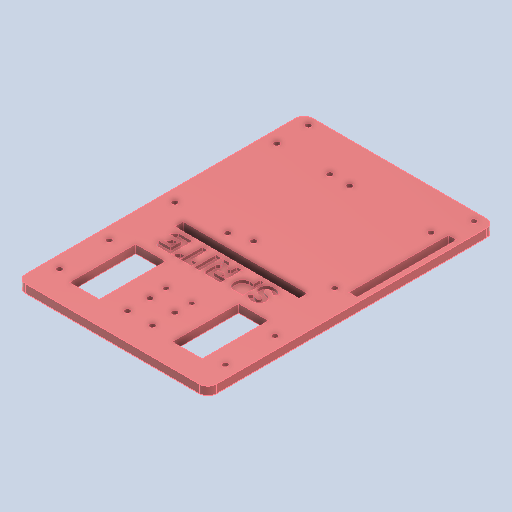
# Autodesk Inventor part: top plate modified
Saved by Autodesk Inventor 2025.1 (Build 291241020, 241B)
## iProperties
Created: 2024-03-20
Part Number: top plate modified
Material: Generic
Document SubType Name: Modeling
Designer: david
Density: 1 g/cm^3
Appearance: Smooth - Red
Description: Top Plate
Author: david
Autodesk Inventor part; units mm, degrees
ref_plane "YZ Plane" through (0, 0, 0) normal (1, 0, 0) x (0, 1, 0)
ref_plane "XZ Plane" through (0, 0, 0) normal (0, 1, 0) x (-1, 0, 0)
ref_plane "XY Plane" through (0, 0, 0) normal (0, 0, 1) x (1, 0, 0)
sketch "Sketch1" plane through (0, 0, 0) normal (0, 1, 0) x (-1, 0, 0)
  line L0 (57.5, -173) -> (57.5, -173) construction
  line L1 (-57.5, -173) -> (-57.5, 0) construction
  line L2 (-57.5, 0) -> (57.5, 0)
  line L3 (57.5, 0) -> (57.5, -173) construction
  line L4 (80.5, 0) -> (-80.5, 0) construction
  line L5 (0, -207.6) -> (0, 34.6) construction
  line L6 (57.5, -173) -> (-57.5, -173)
  line L7 (-57.5, -173) -> (-57.5, -173) construction
  line L8 (57.5, 0) -> (-55.1767, 0)
  line L9 (57.5, -40) -> (-57.5, -40) construction
  line L10 (-57.5, -40) -> (-57.5, 0)
  line L11 (-57.5, 0) -> (57.5, 0)
  line L12 (57.5, 0) -> (57.5, -40)
  line L13 (-57.5, -173) -> (-57.5, -40)
  line L14 (57.5, -173) -> (57.5, -40)
  point P0 (0, 0)
  dimension "width" = 115
  dimension "Length" = 173
  dimension "d2" = 115
  dimension "d112" = 40
  constraints: 26 end point, 6 parallel, 5 horizontal, 4 perpendicular, 1 collinear, 1 point on line, 1 symmetric about line, 1 vertical alignment, 1 other
  measures "width" distance of L1.end L2.end
  measures "Length" distance of L1.start L1.end
  measures "d2" distance of L6.end L0.end
  measures "d112" distance between parallel lines of L2 L9
extrude "Base" add sketch "Sketch1" against normal blind 5
sketch "Sketch11" plane through (0, 0, 0) normal (0, 1, 0) x (1, 0, 0)
  line L0 (0, 207.6) -> (0, -34.6) construction
  line L1 (-57.5, 0) -> (57.5, 0) construction
  line L2 (57.5, 173) -> (-57.5, 173) projected
  line L3 (-50, 18) -> (50, 18) construction
  line L4 (50, 18) -> (50, 48) construction
  line L5 (50, 48) -> (-50, 48) construction
  line L6 (-50, 48) -> (-50, 18) construction
  point P0 (0, 0)
  point P1 (50, 168)
  point P2 (-50, 168)
  dimension "d91" = 18
  dimension "d92" = 50
  dimension "d93" = 5
  dimension "d94" = 50
  dimension "d113" = 30
  constraints: 8 end point, 2 coincident, 2 parallel, 2 symmetric about line, 1 horizontal, 1 perpendicular, 1 vertical alignment
  measures "d91" distance from line of L1 point (50, 18)
  measures "d92" distance from line of point (50, 18) L0
  measures "d93" distance from line of L2 point (50, 168)
  measures "d94" distance from line of L0 point (50, 168)
  measures "d113" distance of L3.end L4.end
hole "Mounting Holes" at (50, 0, -18) at (-50, 0, -18) at (50, 0, -168) at (-50, 0, -168) at (-50, 0, -48) at (50, 0, -48) direction (0, -1, 0) diameter 3.4 depth 6
fillet "Fillet1" radius 5 4 edges at (-57.5, -2.5, 0) (57.5, -2.5, -173) (-57.5, -2.5, -173) (57.5, -2.5, 0)
sketch "Sketch12" plane through (0, 0, 0) normal (0, 1, 0) x (1, 0, 0)
  line L0 (-6, 149) -> (43, 149) construction
  line L1 (43, 149) -> (43, 91) construction
  line L2 (43, 91) -> (-6, 91) construction
  line L3 (-6, 91) -> (-6, 149) construction
  line L4 (-57.5, 168) -> (-57.5, 5) projected
  line L5 (0, 207.6) -> (0, -34.6) projected
  line L6 (-52.5, 0) -> (52.5, 0) projected
  circle A0 centre (-50, 48) radius 1.7 projected
  line L7 (52.5, 173) -> (-52.5, 173) projected
  circle A1 centre (50, 48) radius 1.7 projected
  circle A2 centre (50, 168) radius 1.7 projected
  point P0 (0, 0)
  point P1 (0, 0)
  point P2 (52.2987, 0)
  point P3 (-57.5, 40)
  point P4 (0, 0)
  dimension "d104" = 58
  dimension "d263" = 24
  dimension "d266" = 49
  dimension "d267" = 7
  constraints: 8 end point, 1 horizontal, 1 midpoint, 1 parallel, 1 perpendicular, 1 vertical
  measures "d104" distance of L0.end L1.end
  measures "d263" distance between parallel lines of L7 L0
  measures "d266" distance of L1.end L2.end
  measures "d267" distance from line of L1 A2.centre
hole "RasPi Mounting Holes" at (-6, 0, -149) at (43, 0, -149) at (43, 0, -91) at (-6, 0, -91) direction (0, -1, 0) diameter 3.4 depth 6
sketch "Sketch15" plane through (0, 0, 0) normal (0, 1, 0) x (1, 0, 0)
  line L0 (-18, 149) -> (-18, 87.5) construction
  line L1 (-18, 87.5) -> (-50, 87.5) construction
  line L2 (-50, 87.5) -> (-50, 149) construction
  line L3 (-50, 149) -> (-18, 149) construction
  line L4 (-52.5, 0) -> (52.5, 0) projected
  circle A0 centre (43, 149) radius 1.7 projected
  circle A1 centre (50, 48) radius 1.7 projected
  circle A2 centre (-50, 48) radius 1.7 projected
  point P0 (0, 0)
  point P1 (0, 0)
  dimension "d122" = 32
  dimension "d123" = 61.5
  constraints: 8 end point, 4 coincident, 2 parallel, 1 horizontal alignment, 1 midpoint, 1 perpendicular, 1 vertical, 1 vertical alignment
  measures "d122" distance of L2.end L0.start
  measures "d123" distance of L1.end L2.end
hole "LM2596 Mounting Holes" at (-18, 0, -149) at (-18, 0, -87.5) at (-50, 0, -87.5) at (-50, 0, -149) direction (0, -1, 0) diameter 3.4 depth 6
sketch "Sketch16" plane through (0, 0, 0) normal (0, 1, 0) x (1, 0, 0)
  line L0 (-7.5, 16.5) -> (7.5, 16.5) construction
  line L1 (7.5, 16.5) -> (7.5, 30) construction
  line L2 (7.5, 30) -> (-7.5, 30) construction
  line L3 (-7.5, 30) -> (-7.5, 16.5) construction
  line L4 (52.5, 173) -> (-52.5, 173) projected
  line L5 (-52.5, 0) -> (52.5, 0) projected
  point P0 (0, 0)
  point P1 (0, 30)
  point P2 (0, 173)
  dimension "d132" = 15
  dimension "d133" = 13.5
  dimension "d264" = 16.5
  constraints: 8 end point, 4 coincident, 2 midpoint, 2 parallel, 1 horizontal, 1 perpendicular, 1 vertical alignment
  measures "d132" distance of L1.end L2.end
  measures "d133" distance of L2.end L0.start
  measures "d264" distance from line of L5 point (7.5, 16.5)
hole "Camera Mount Mounting Holes" at (-7.5, 0, -30) at (-7.5, 0, -16.5) at (7.5, 0, -16.5) at (7.5, 0, -30) direction (0, -1, 0) diameter 3.4 depth 6
sketch "Sketch17" plane through (0, 0, 0) normal (0, 1, 0) x (1, 0, 0)
  spline S0 degree 4 poles (20.2958, 60.9862) (20.6789, 60.4096) (23.4396, 59.0106) (25.9197, 59.115) (27.89, 60.1434) (29.1867, 61.8157) (29.4113, 63.6805) (28.5047, 66.7307) (25.5201, 67.2591) (20.7186, 68.3485) (23.8724, 71.7602) (26.3838, 70.0239) (28.1257, 68.7657) knots 0 0 0 0 0 0.20272 0.281355 0.355202 0.433006 0.519581 0.610324 0.697239 0.780232 1 1 1 1 1
  line L0 (28.1257, 68.7657) -> (29.7111, 70.7885)
  line L1 (20.2958, 60.9862) -> (21.6797, 63.1653)
  spline S1 degree 4 poles (21.6797, 63.1653) (22.294, 62.9002) (22.8002, 62.0758) (25.5673, 61.3366) (26.8616, 62.9242) (26.2496, 64.3208) (24.0458, 64.6545) (23.329, 64.9908) (21.3928, 65.6303) (20.3004, 66.9273) (19.7305, 68.0113) (20.0556, 71.293) (23.128, 73.4529) (27.765, 72.9465) (29.2945, 71.0114) (29.7111, 70.7885) knots 0 0 0 0 0 0.144957 0.205265 0.266901 0.324627 0.385746 0.449033 0.509009 0.575778 0.647334 0.728378 0.816758 1 1 1 1 1
  line L2 (19.0392, 59.5823) -> (19.0392, 72.6249)
  line L3 (19.0392, 72.6249) -> (16.3103, 72.6177)
  line L4 (16.3103, 72.6177) -> (16.3103, 68.7657)
  line L5 (16.3005, 62.1221) -> (16.3005, 66.1835)
  line L6 (16.3005, 66.1835) -> (13.9834, 66.1835)
  line L7 (16.3005, 62.1221) -> (13.9834, 62.1221)
  line L8 (19.0392, 59.5823) -> (13.9055, 59.5823)
  line L9 (16.3103, 68.7657) -> (13.9055, 68.7657)
  spline S2 degree 4 poles (13.9055, 59.5823) (12.4366, 59.3633) (9.7113, 60.1855) (9.0071, 64.9843) (10.0268, 67.2624) (11.8162, 68.8385) (13.9055, 68.7657) knots 0 0 0 0 0 0.424491 0.584677 1 1 1 1 1
  spline S3 degree 4 poles (13.9834, 62.1221) (12.4908, 61.883) (10.9878, 63.9228) (12.1538, 66.1308) (13.9834, 66.1835) knots 0 0 0 0 0 1 1 1 1 1
  line L10 (5.611, 63.3617) -> (5.611, 72.6389)
  line L11 (5.611, 72.6389) -> (2.2951, 72.6389)
  line L12 (2.2951, 72.6389) -> (2.2951, 72.4635)
  line L13 (2.2951, 72.4635) -> (2.2951, 68.7172)
  line L14 (2.2951, 68.7172) -> (0.5839, 68.7172)
  line L15 (0.5839, 68.7172) -> (-1.936, 72.6389)
  line L16 (-1.936, 72.6389) -> (-5.9376, 72.6389)
  line L17 (-5.9376, 72.6389) -> (-3.4177, 68.7172)
  line L18 (5.611, 63.3617) -> (2.2951, 63.3617)
  line L19 (2.2951, 63.3617) -> (2.2951, 65.3318)
  line L20 (2.2951, 65.3318) -> (-1.6405, 65.3318)
  line L21 (-1.6405, 65.3318) -> (-1.6405, 62.7426)
  line L22 (-1.6405, 62.7426) -> (5.611, 62.7426)
  line L23 (5.611, 62.7426) -> (5.611, 59.4347)
  line L24 (5.611, 59.4347) -> (-3.7057, 59.4347)
  line L25 (-5.0121, 60.8841) -> (-5.0121, 67.0542)
  arc A0 (-3.4177, 68.7172) -> (-5.0121, 67.0542) centre (-3.281, 66.9903) ccw
  arc A1 (-5.0121, 60.8841) -> (-3.7057, 59.4347) centre (-2.6718, 61.68) ccw
  line L26 (-6.9039, 59.4347) -> (-10.2687, 59.4347)
  line L27 (-10.2687, 59.4347) -> (-10.2687, 72.6389)
  line L28 (-10.2687, 72.6389) -> (-6.9039, 72.6389)
  line L29 (-6.9039, 72.6389) -> (-6.9039, 59.4347)
  line L30 (-11.8026, 59.4347) -> (-11.8026, 62.7426)
  line L31 (-11.8026, 62.7426) -> (-15.1713, 62.7426)
  line L32 (-15.1713, 62.7426) -> (-15.1713, 72.6389)
  line L33 (-15.1713, 72.6389) -> (-18.4823, 72.6389)
  line L34 (-18.4823, 72.6389) -> (-18.4823, 59.4347)
  line L35 (-18.4823, 59.4347) -> (-11.8026, 59.4347)
  line L36 (-19.0962, 59.4347) -> (-19.0962, 62.7426)
  line L37 (-19.0962, 62.7426) -> (-21.5406, 62.7426)
  line L38 (-21.5406, 62.7426) -> (-23.787, 59.4347)
  line L39 (-23.787, 59.4347) -> (-19.0962, 59.4347)
  line L40 (-24.4617, 59.4285) -> (-24.4617, 72.6389)
  line L41 (-24.4617, 72.6389) -> (-27.7836, 72.6389)
  line L42 (-27.7836, 72.6389) -> (-27.7836, 59.4285)
  line L43 (-27.7836, 59.4285) -> (-24.4617, 59.4285)
  line L44 (-28.3589, 64.3467) -> (-28.3589, 67.6986)
  line L45 (-28.3589, 67.6986) -> (-30.851, 67.6986)
  line L46 (-30.851, 64.3467) -> (-28.3589, 64.3467)
  line L47 (-27.7836, 59.4285) -> (-27.7836, 62.7665)
  line L48 (-27.7836, 62.7665) -> (-32.8922, 62.7665)
  line L49 (-32.8922, 59.4285) -> (-27.7836, 59.4285)
  line L50 (-32.8922, 59.4285) -> (-35.0606, 62.7665)
  line L51 (-35.0606, 62.7665) -> (-32.8922, 62.7665)
  line L52 (-30.851, 64.3467) -> (-33.0635, 64.3745)
  line L53 (-33.0635, 64.3745) -> (-30.851, 67.6986)
  line L54 (-27.7836, 69.2996) -> (-35.0607, 69.2996)
  line L55 (-35.0607, 69.2996) -> (-32.8922, 72.6389)
  line L56 (-32.8922, 72.6389) -> (-27.7836, 72.6389)
  point P0 (21.8312, 59.9838)
  point P1 (24.6762, 59.2804)
  point P2 (27.8239, 60.2947)
  point P3 (29.2122, 63.5388)
  point P4 (25.048, 67.3986)
  point P5 (22.697, 68.6)
  point P6 (22.9251, 69.7776)
  point P7 (24.696, 70.4127)
  point P8 (28.2025, 66.0753)
  point P9 (28.8947, 61.6912)
  point P10 (26.5311, 59.549)
  point P11 (22.4682, 62.66)
  point P12 (23.9337, 61.9871)
  point P13 (25.8462, 62.0797)
  point P14 (26.5371, 62.9822)
  point P15 (26.0534, 64.0216)
  point P16 (24.2764, 64.6696)
  point P17 (23.1794, 65.02)
  point P18 (21.5575, 65.763)
  point P19 (20.447, 66.8371)
  point P20 (19.9672, 67.9776)
  point P21 (20.2871, 70.5583)
  point P22 (22.4689, 72.5357)
  point P23 (26.4542, 72.6342)
  point P24 (29.0183, 71.3375)
  point P25 (11.42, 60.0557)
  point P26 (9.7835, 62.015)
  point P27 (9.4634, 64.5517)
  point P28 (9.8877, 66.3528)
  point P29 (11.0438, 67.8413)
  point P30 (12.7043, 62.5399)
  point P31 (12.0389, 63.8771)
  point P32 (12.4464, 65.3868)
  point P33 (-27.7836, 62.7665)
  point P34 (-3.281, 66.9903)
  constraints: 114 end point, 8 point on line, 4 point on circle, 2 centre point, 41 other
extrude "SP RITE Logo" cut sketch "Sketch17" against normal blind 2 contours L1 S1 L0 S0 | L8 S2 L9 L4 L3 L2 | L7 S3 L6 L5 | L18 L19 L20 L21 L22 L23 L24 A1 L25 A0 L17 L16 L15 L14 L13 L12 L11 L10 | L26 L27 L28 L29 | L35 L34 L33 L32 L31 L30 | L39 L38 L37 L36 | L43 L42 L41 L40 | L49 L50 L51 L48 L42 | L42 L54 L55 L56 | L46 L52 L53 L45 L44
sketch "Sketch18" plane through (0, 0, 0) normal (0, 1, 0) x (1, 0, 0)
  line L0 (40, 14) -> (22, 14)
  line L1 (22, 14) -> (22, 54)
  line L2 (22, 54) -> (40, 54)
  line L3 (40, 54) -> (40, 14)
  line L4 (-52.5, 0) -> (52.5, 0) projected
  line L5 (49.5, 93) -> (54.5, 93)
  line L6 (54.5, 93) -> (54.5, 153)
  line L7 (54.5, 153) -> (49.5, 153)
  line L8 (49.5, 153) -> (49.5, 93)
  line L9 (57.5, 5) -> (57.5, 168) projected
  line L10 (52.5, 173) -> (-52.5, 173) projected
  line L11 (37.5, 75) -> (-37.5, 75)
  line L12 (-37.5, 75) -> (-37.5, 80)
  line L13 (-37.5, 80) -> (37.5, 80)
  line L14 (37.5, 80) -> (37.5, 75)
  line L15 (0, 0) -> (0, 173) construction
  line L16 (-40, 14) -> (-22, 14)
  line L17 (-22, 14) -> (-22, 54)
  line L18 (-22, 54) -> (-40, 54)
  line L19 (-40, 54) -> (-40, 14)
  circle A0 centre (-7.78, 65) radius 1.56
  circle A1 centre (7.78, 65) radius 1.56
  point P0 (0, 0)
  point P1 (22, 34)
  point P2 (0, 75)
  dimension "d268" = 40
  dimension "d269" = 18
  dimension "d270" = 22
  dimension "d271" = 14
  dimension "d272" = 5
  dimension "d273" = 3
  dimension "d274" = 60
  dimension "d275" = 20
  dimension "d276" = 75
  dimension "d277" = 5
  dimension "d278" = 75
  dimension "d279" = 15.56
  dimension "d280" = 7.78
  dimension "d281" = 65
  dimension "d282" = 3.12
  constraints: 34 end point, 6 midpoint, 6 parallel, 4 symmetric about line, 3 horizontal, 3 perpendicular, 2 centre point, 1 equal radius, 1 horizontal alignment, 1 vertical alignment
  measures "d268" distance of L2.end L0.start
  measures "d269" distance of L0.start L0.end
  measures "d270" horizontal distance of point (0, 0) point (22, 34)
  measures "d271" distance between parallel lines of L4 L0
  measures "d272" distance of L6.end L7.end
  measures "d273" distance between parallel lines of L9 L6
  measures "d274" distance of L5.end L6.end
  measures "d275" distance between parallel lines of L10 L7
  measures "d276" distance between parallel lines of L4 L11
  measures "d277" distance of L11.end L12.end
  measures "d278" distance of L11.start L11.end
  measures "d279" distance of A0.centre A1.centre
  measures "d280" horizontal distance of A0.centre point (0, 0)
  measures "d281" distance from line of L4 A0.centre
  measures "d282" diameter of A0
extrude "Extrusion6" cut sketch "Sketch18" against normal blind 10 contours L0 L1 L2 L3 | L8 L7 L6 L5 | L11 L12 L13 L14 | L19 L18 L17 L16
sketch "Sketch19" plane through (0, 0, 0) normal (0, 1, 0) x (1, 0, 0)
  line L0 (-37.5, 75) -> (-37.5, 80) projected
  line L1 (-37.5, 80) -> (37.5, 80) projected
  line L2 (37.5, 80) -> (37.5, 75) projected
  line L3 (37.5, 75) -> (-37.5, 75) projected
  line L4 (-40, 54) -> (-22, 54) projected
  line L5 (-22, 54) -> (-22, 14) projected
  line L6 (-22, 14) -> (-40, 14) projected
  line L7 (-40, 14) -> (-40, 54) projected
  line L8 (49.5, 153) -> (54.5, 153) projected
  line L9 (54.5, 153) -> (54.5, 93) projected
  line L10 (54.5, 93) -> (49.5, 93) projected
  line L11 (49.5, 93) -> (49.5, 153) projected
  line L12 (22, 14) -> (22, 54) projected
  line L13 (22, 54) -> (40, 54) projected
  line L14 (40, 54) -> (40, 14) projected
  line L15 (40, 14) -> (22, 14) projected
  line L16 (-10.2687, 59.4347) -> (-10.2687, 72.6389) projected
  line L17 (-10.2687, 72.6389) -> (-6.9039, 72.6389) projected
  line L18 (-6.9039, 72.6389) -> (-6.9039, 59.4347) projected
  line L19 (-6.9039, 59.4347) -> (-10.2687, 59.4347) projected
  line L20 (-28.3589, 64.3467) -> (-30.851, 64.3467) projected
  line L21 (-30.851, 64.3467) -> (-33.0635, 64.3745) projected
  line L22 (-33.0635, 64.3745) -> (-30.851, 67.6986) projected
  line L23 (-30.851, 67.6986) -> (-28.3589, 67.6986) projected
  line L24 (-28.3589, 67.6986) -> (-28.3589, 64.3467) projected
  line L25 (-15.1713, 72.6389) -> (-15.1713, 62.7426) projected
  line L26 (-15.1713, 62.7426) -> (-11.8026, 62.7426) projected
  line L27 (-11.8026, 62.7426) -> (-11.8026, 59.4347) projected
  line L28 (-11.8026, 59.4347) -> (-18.4823, 59.4347) projected
  line L29 (-18.4823, 59.4347) -> (-18.4823, 72.6389) projected
  line L30 (-18.4823, 72.6389) -> (-15.1713, 72.6389) projected
  line L31 (29.7111, 70.7885) -> (28.1257, 68.7657) projected
  line L32 (20.2958, 60.9862) -> (21.6797, 63.1653) projected
  line L33 (2.2951, 72.6389) -> (5.611, 72.6389) projected
  line L34 (5.611, 72.6389) -> (5.611, 63.3617) projected
  line L35 (5.611, 63.3617) -> (2.2951, 63.3617) projected
  line L36 (2.2951, 63.3617) -> (2.2951, 65.3318) projected
  line L37 (2.2951, 65.3318) -> (-1.6405, 65.3318) projected
  line L38 (-1.6405, 65.3318) -> (-1.6405, 62.7426) projected
  line L39 (-1.6405, 62.7426) -> (5.611, 62.7426) projected
  line L40 (5.611, 62.7426) -> (5.611, 59.4347) projected
  line L41 (5.611, 59.4347) -> (-3.7057, 59.4347) projected
  arc A0 (-5.0121, 60.8841) -> (-3.7057, 59.4347) centre (-2.6718, 61.68) ccw projected
  line L42 (-5.0121, 60.8841) -> (-5.0121, 67.0542) projected
  arc A1 (-3.4177, 68.7172) -> (-5.0121, 67.0542) centre (-3.281, 66.9903) ccw projected
  line L43 (-3.4177, 68.7172) -> (-5.9376, 72.6389) projected
  line L44 (-5.9376, 72.6389) -> (-1.936, 72.6389) projected
  line L45 (-1.936, 72.6389) -> (0.5839, 68.7172) projected
  line L46 (0.5839, 68.7172) -> (2.2951, 68.7172) projected
  line L47 (2.2951, 68.7172) -> (2.2951, 72.6389) projected
  line L48 (-35.0607, 69.2996) -> (-32.8922, 72.6389) projected
  line L49 (-32.8922, 72.6389) -> (-24.4617, 72.6389) projected
  line L50 (-24.4617, 72.6389) -> (-24.4617, 59.4285) projected
  line L51 (-24.4617, 59.4285) -> (-32.8922, 59.4285) projected
  line L52 (-32.8922, 59.4285) -> (-35.0606, 62.7665) projected
  line L53 (-35.0606, 62.7665) -> (-27.7836, 62.7665) projected
  line L54 (-27.7836, 62.7665) -> (-27.7836, 69.2996) projected
  line L55 (-27.7836, 69.2996) -> (-35.0607, 69.2996) projected
  line L56 (-23.787, 59.4347) -> (-21.5406, 62.7426) projected
  line L57 (-21.5406, 62.7426) -> (-19.0962, 62.7426) projected
  line L58 (-19.0962, 62.7426) -> (-19.0962, 59.4347) projected
  line L59 (-19.0962, 59.4347) -> (-23.787, 59.4347) projected
  line L60 (16.3103, 72.6177) -> (19.0392, 72.6249) projected
  line L61 (19.0392, 72.6249) -> (19.0392, 59.5823) projected
  line L62 (19.0392, 59.5823) -> (13.9055, 59.5823) projected
  line L63 (13.9055, 68.7657) -> (16.3103, 68.7657) projected
  line L64 (16.3103, 68.7657) -> (16.3103, 72.6177) projected
  circle A2 centre (7.5, 16.5) radius 1.7 projected
  circle A3 centre (-7.5, 30) radius 1.7 projected
  circle A4 centre (-7.5, 16.5) radius 1.7 projected
  circle A5 centre (7.5, 30) radius 1.7 projected
  circle A6 centre (-50, 87.5) radius 1.7 projected
  circle A7 centre (-18, 149) radius 1.7 projected
  circle A8 centre (-18, 87.5) radius 1.7 projected
  circle A9 centre (-50, 149) radius 1.7 projected
  circle A10 centre (43, 91) radius 1.7 projected
  circle A11 centre (-6, 149) radius 1.7 projected
  circle A12 centre (43, 149) radius 1.7 projected
  circle A13 centre (-6, 91) radius 1.7 projected
  circle A14 centre (-50, 48) radius 1.7 projected
  circle A15 centre (50, 168) radius 1.7 projected
  circle A16 centre (50, 18) radius 1.7 projected
  circle A17 centre (-50, 18) radius 1.7 projected
  circle A18 centre (-50, 168) radius 1.7 projected
  circle A19 centre (50, 48) radius 1.7 projected
  arc A20 (52.5, 0) -> (57.5, 5) centre (52.5, 5) ccw projected
  line L65 (57.5, 5) -> (57.5, 168) projected
  arc A21 (57.5, 168) -> (52.5, 173) centre (52.5, 168) ccw projected
  line L66 (52.5, 173) -> (-52.5, 173) projected
  arc A22 (-52.5, 173) -> (-57.5, 168) centre (-52.5, 168) ccw projected
  line L67 (-57.5, 168) -> (-57.5, 5) projected
  arc A23 (-57.5, 5) -> (-52.5, 0) centre (-52.5, 5) ccw projected
  line L68 (-52.5, 0) -> (52.5, 0) projected
  line L69 (0, 209.0497) -> (0, -36.0497) projected
  point P0 (0, 0)
  point P1 (-7.78, 40)
  point P2 (7.78, 40)
  dimension "d285" = 15.56
  dimension "d286" = 10
  constraints: 1 horizontal alignment, 1 symmetric about line, 1 vertical alignment, 2 other
  measures "d285" distance of point (-7.78, 40) point (7.78, 40)
  measures "d286" vertical distance of point (-7.78, 40) A3.centre
hole "Hole11" at (-7.78, 0, -40) at (7.78, 0, -40) direction (0, -1, 0) diameter 3 end through all
equation "\"d2\" = width"
equation "\"d94\" = d92"
equation "\"d95\" = HoleDia"
equation "\"d105\" = HoleDia"
equation "\"d125\" = HoleDia"
equation "\"d135\" = HoleDia"
equation "\"d280\" = 0.5 * d279"
equation "\"HoleDia\" = 3.4"
body "Solid1"
